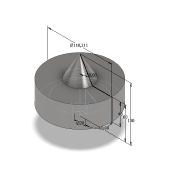
# Autodesk Inventor part: Mass_otimization
Saved by Autodesk Inventor 2021 (Build 250183000, 183)
## iProperties
RuleStatus: InUse
Created: 2025-08-13
Part Number: Mass_otimization
Material: Steel, Mild
Document SubType Name: Modeling
Designer: RAFAEL
Density: 7.85 g/cm^3
Appearance: Semi-Polished
Mass: 3000 g
Surface Area: 412.685 cm^2
Volume: 382.166 cm^3
Author: RAFAEL
Autodesk Inventor part; units mm, degrees
note: some values were not read from the file. Left out: dimensions or parameters whose unit could not be read.
ref_plane "YZ Plane" through (0, 0, 0) normal (1, 0, 0) x (0, 1, 0)
ref_plane "XZ Plane" through (0, 0, 0) normal (0, 1, 0) x (-1, 0, 0)
ref_plane "XY Plane" through (0, 0, 0) normal (0, 0, 1) x (1, 0, 0)
sketch "Sketch1" plane through (0, 0, 0) normal (0, 0, 1) x (1, 0, 0)
  line L0 (0, 0) -> (10, 0)
  line L1 (10, 0) -> (10, 48.3509)
  line L2 (10, 48.3509) -> (59.1053, 20)
  line L3 (59.1053, 20) -> (59.1053, 60)
  line L4 (59.1053, 60) -> (23.094, 60)
  line L5 (23.094, 60) -> (0, 100)
  line L6 (0, 100) -> (0, 0)
  dimension "d0" = 20
  dimension "d1" = 30
  dimension "d2" = 100
  dimension "d3" = 60
  dimension "d4" = 40
  dimension "d5" = 118.2105
  dimension "d6" = 60
  constraints: 15 end point, 2 horizontal, 2 perpendicular, 1 parallel
  measures "d0" diameter of L1 L6
  measures "d1" angle of L5 L6
  measures "d2" distance of L0.start L5.end
  measures "d3" angle of L2 L1
  measures "d4" distance of L2.end L3.end
  measures "d5" diameter of L3 L6
  measures "d6" distance from line of L4 L0.end
revolve "Revolution1" add sketch "Sketch1" angle 360 about axis through (0, 100, 0) along (0, -1, 0)
fillet "Fillet1" radius 20 1 edges at (-10, 48.3509, 0)
equation "\"ITERACOES\" = 0"
equation "\"VALORES_OTIMOS\" = 118.21054"
body "Solid1"
